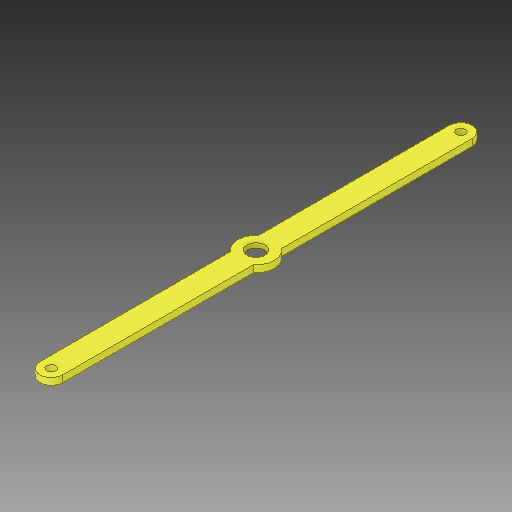
# Autodesk Inventor part: 04-02-Тяга
Saved by Autodesk Inventor 2018 (Build 220112000, 112)
## iProperties
Part Number: 04-02-Тяга
Material: Типовые
Document SubType Name: Modeling
Designer: sbnnl
Density: 1 g/cm^3
Appearance: Гладкий - желтый
Author: sbnnl
Autodesk Inventor part; units mm, degrees
ref_plane "YZ Plane" through (0, 0, 0) normal (1, 0, 0) x (0, 1, 0)
ref_plane "XZ Plane" through (0, 0, 0) normal (0, 1, 0) x (-1, 0, 0)
ref_plane "XY Plane" through (0, 0, 0) normal (0, 0, 1) x (1, 0, 0)
sketch "Эскиз1" plane through (0, 0, 0) normal (0, 1, 0) x (-1, 0, 0)
  circle A0 centre (0, 0) radius 2
  line L0 (0, 0) -> (0, -180) construction
  circle A1 centre (0, -180) radius 2
  arc A2 (5, 0) -> (-5, 0) centre (0, 0) ccw
  arc A3 (-5, -180) -> (5, -180) centre (0, -180) ccw
  line L1 (5, -180) -> (5, -96.245)
  line L2 (-5, -180) -> (-5, -96.245)
  line L3 (0, -90) -> (22.1641, -90) construction
  line L4 (5, -83.755) -> (5, 0)
  line L5 (-5, -83.755) -> (-5, 0)
  arc A4 (-5, -83.755) -> (-5, -96.245) centre (0, -90) ccw
  arc A5 (5, -96.245) -> (5, -83.755) centre (0, -90) ccw
  circle A6 centre (0, -90) radius 4
  dimension "d0" = 4
  dimension "d1" = 4
  dimension "d2" = 180
  dimension "d3" = 10
  dimension "d4" = 10
  dimension "d8" = 8
  dimension "d9" = 8
  constraints: 12 end point, 8 point on circle, 7 centre point, 6 coincident, 5 vertical, 4 tangent, 1 concentric, 1 horizontal, 1 midpoint
  measures "d0" diameter of A0
  measures "d1" diameter of A1
  measures "d2" distance of L0.start L0.end
  measures "d3" diameter of A2
  measures "d4" diameter of A3
  measures "d8" radius of A5
  measures "d9" diameter of A6
extrude "Выдавливание1" add sketch "Эскиз1" along normal blind 3
sketch "Эскиз2" plane through (0, 0, 0) normal (0, -1, 0) x (1, 0, 0)
  circle A0 centre (0, 0) radius 3.5
  circle A1 centre (0, -180) radius 2 projected
  circle A2 centre (0, -180) radius 3.5
  circle A3 centre (0, 0) radius 2 projected
  dimension "d10" = 7
  dimension "d11" = 7
  constraints: 2 centre point, 2 coincident
  measures "d10" diameter of A0
  measures "d11" diameter of A2
extrude "Выдавливание2" add sketch "Эскиз2" along normal blind 1.5
chamfer "Фаска1" distance 1.2 angle 45 2 edges at (-3.5, -1.5, 0) (-3.5, -1.5, -180)
sketch "Эскиз3" plane through (0, 0, 0) normal (0, -1, 0) x (1, 0, 0)
  circle A0 centre (0, -90) radius 4 projected
  circle A1 centre (0, -90) radius 5
  point P0 (0, 0)
  dimension "d17" = 10
  constraints: 1 centre point, 1 coincident
  measures "d17" diameter of A1
extrude "Выдавливание3" cut sketch "Эскиз3" against normal blind 1
